Autodesk Fusion 360 part; units mm, degrees
(part 3 of 3)
extrude "Extruir16" cut sketch "Boceto24" against normal blind 2 contours L4 L5 L6 L7 L8 L9 L10 L11 L12 L13 L14 L15 L16 L17 L18 L19 L20 L21 L22 L23 L24 L25 L26 L27 L28 L29 L30 L31 L32 L33 L34 L35 L36 L37 L38 L39 L40 L41 L42 L43 L44 L45 L46 L47 L48 L49 L50 L51 L52 L53 L54 L55 L56 L57 L58 L59 L60 L61 L62 L63 L64 L65 L66 L67 L68 L69 L70 L71 L72 L73 L74 L75 L76 L77 L78 L79 L80 L81 L82 L83 L84 L85 L86 L87 L88 L89 L90 L91 L92 L93 L94 L95 L96 L97 L98 L99 L100 L101 L102 L103 L104 L105 L106 L107 L108 L109 L110 L111 L112 L113 L114 L115 L116 L117 L118 L119 L120 L121 L122 L123 L124 L125 L126 L127 L128 L129 L130 L131 L132 L133 L134 L135 L136 L137 L138 L139 L140 L141 L142 L143 L144 L145 L146 L147 L148 L149 L150 L151 L152 L153 L154 L155 L156 L157 L158 L159 L160 L161 L162 L163 L164 L165 L166 L167 L168 L169 L170 L171 L172 L173 L174 L175 L176 L177 L178 L179 L180 L181 L182 L183 L184 L185 L186 L187 L188 L189 L190 L191 L192 L193 L194 L195 L196 L197 L198 L199 L200 L201 L202 L203 L204 L205 L206 L207 L208 L209 L210 L211 L212 L213 L214 L215 L216 L217 L218 L219 L220 L221 L222 L223 L224 L225 L226 L227 L228 L229 L230 L231 L232 L233 L234 L235 L236 L237 L238 L239 L240 L241 L242 L243 L244 L245 L246 L247 L248 L249 L250 L251 L252 L253 L254 L255 L256 L257 L258 L259 L260 L261 L262 L263 L264 L265 L266 L267 L268 L269 L270 L271 L272 L273 L274 L275 L276 L277 L278 L279 L280 L281 L282 L283 L284 L285 L286 L287 | L288 L289 L290 L291 L292 L293 L294 L295 L296 L297 L298 L299 L300 L301 L302 L303 L304 L305 L306 L307 L308 L309 L310 L311 L312 L313 L314 L315 L316 L317 L318 L319 L320 L321 L322 L323 L324 L325 L326 L327 L328 L329 L330 L331 L332 L333 L334 L335 L336 L337 L338 L339 L340 L341 L342 L343 L344 | L345 L346 L347 L348 L349 L350 L351 L352 L353 L354 L355 L356 L357 L358 L359 L360 L361 L362 L363 L364 L365 L366 L367 L368 L369 L370 L371 L372 L373 L374 L375 L376 L377 L378 L379 L380 L381 L382 L383 L384 L385 L386 L387 L388 L389 L390 L391 L392 L393 L394 L395 L396 L397 L398 L399 L400 L401 L402 L403 L404 L405 L406 L407 L408 L409 L410 L411 L412 L413 L414 L415 L416 L417 L418 L419 L420 L421 L422 L423 L424 L425 L426 L427 L428 L429 L430 L431 L432 L433 L434 L435 L436 L437 L438 L439 L440 L441 L442 L443 L444 L445 L446 L447 | L448 L449 L450 L451 L452 L453 L454 L455 L456 L457 L458 L459 L460 L461 L462 L463 L464 L465 L466 L467 L468 L469 L470 L471 L472 L473 L474 L475 L476 L477 L478 L479 L480 L481 L482 L483 L484 L485 L486 L487 L488 L489 L490 L491 L492 L493 L494 L495 L496 L497 L498 L499 L500 L501 L502 L503 L504 L505 L506 L507 L508 L509 L510 L511 L512 L513 L514 L515 L516 L517 L518 L519 L520 L521 L522 L523 L524 L525 L526 L527 L528 L529 L530 L531 L532 L533 L534 L535 L536 L537 L538 L539 L540 L541 L542 L543 L544 L545 L546 L547 L548 L549 L550 | L551 L552 L553 L554 L555 L556 L557 L558 L560 L561 L562 L563 L564 L565 L566 L567 L569 L570 L571 L572 L573 L575 L576 L577 L579 L580 L581 L583 L584 L585 L586 L587 L588 L589 L590 L591 L592 L593 L594 L595 L596 L597 L598 L599 L600 L601 L602 L603 L604 L605 L606 L607 L608 L609 L610 L611 L612 L613 L614 L616 L617 L618 L619 L620 L621 L622 L623 L625 L626 L627 L628 L629 L630 L631 L632 L634 L635 L636 L637 L638 L639 L640 L641 L642 L643 L688 L690 L691 L692 L696 L697 L698 L699 L700 L701 L702 L703 L704 L705 L707 L708 L709 L710 L711 L712 L714 L715 L716 L717 L718 L719 L720 L721 L722 L723 L725 L726 L727 L728 L729 L730 L731 L732 L733 L734 L735 L738 L739 L740 L741 L742 L743 L744 L745 L746 L747 L748 L749 L750 L751 L752 L753 L754 L755 L756 L757 L758 L759 L760 L761 L762 L763 L765 L766 L767 L769 L770 L771 L773 L774 L775 L776 L777 L778 L779 L781 L783 | L784 L785 L786 L787 L788 L789 L790 L791 L792 L793 L794 L795 L796 L797 L798 L799 L800 L801 L802 L803 L804 L805 L806 L807 L808 L809 L810 L811 L812 L813 L814 L815 L816 L817 L818 L819 L820 L821 L822 L823 L824 L825 L826 L827 L828 L829 L830 L831 L832 L833 L834 L835 L836 L837 L838 L839 bodies 3
ref_plane "PlanoDeObra7" through (97, 32.5, 92.5) normal (1, 0, 0) x (0, 1, 0)
sketch "Boceto29" plane through (0, -6, 0) normal (0, -1, 0) x (1, 0, 0)
  line L0 (25, 74.5) -> (90, 74.5)
  line L1 (90, 74.5) -> (90, 110.5)
  line L2 (90, 110.5) -> (25, 110.5)
  line L3 (25, 110.5) -> (25, 74.5)
  line L4 (32, 82.5) -> (62, 82.5)
  line L5 (62, 82.5) -> (62, 78.5)
  line L6 (62, 78.5) -> (32, 78.5)
  line L7 (32, 78.5) -> (32, 82.5)
  line L8 (19, 74.5) -> (19, 110.5)
  line L9 (74.5, 90.5) -> (84.5, 90.5)
  line L10 (84.5, 90.5) -> (84.5, 84.5)
  line L11 (84.5, 84.5) -> (74.5, 84.5)
  line L12 (74.5, 84.5) -> (74.5, 90.5)
  line L13 (96, 74.5) -> (96, 110.5)
  line L14 (81, 82.5) -> (88, 82.5)
  line L15 (88, 82.5) -> (88, 75.5)
  line L16 (88, 75.5) -> (81, 75.5)
  line L17 (81, 75.5) -> (81, 82.5)
  dimension "d144" = 13
  dimension "d145" = 30
  dimension "d146" = 4
  dimension "d147" = 4
  dimension "d148" = 10
  dimension "d149" = 6
  dimension "d150" = 20
  dimension "d151" = 11.5
  dimension "d152" = 7
  dimension "d153" = 7
  dimension "d154" = 28
  dimension "d155" = 8
  constraint horizontal L4
  constraint vertical L5
  constraint horizontal L6
  constraint vertical L7
  constraint horizontal L9
  constraint vertical L10
  constraint horizontal L11
  constraint vertical L12
  constraint horizontal L14
  constraint vertical L15
  constraint horizontal L16
  constraint vertical L17
  measures "d144" distance of L7 L8
  measures "d145" distance of L4.start L4.end
  measures "d146" distance of L0 L6
  measures "d147" distance of L4.end L5.end
  measures "d148" distance of L9.start L9.end
  measures "d149" distance of L9.start L11.end
  measures "d150" distance of L2 L9
  measures "d151" distance of L10 L13
  measures "d152" distance of L14.start L14.end
  measures "d153" distance of L14.start L16.end
  measures "d154" distance of L2 L14
  measures "d155" distance of L13 L15
extrude "Extruir21" cut sketch "Boceto29" against normal blind 4 contours L4 L5 L6 L7 | L9 L10 L11 L12 | L14 L15 L16 L17 bodies 3
sketch "Boceto30" plane through (0, 71, 0) normal (0, 1, 0) x (-1, 0, 0)
  line L0 (-90, 74.5) -> (-25, 74.5)
  line L1 (-25, 74.5) -> (-25, 110.5)
  line L2 (-25, 110.5) -> (-90, 110.5)
  line L3 (-90, 110.5) -> (-90, 74.5)
  line L4 (-77, 87.5) -> (-27, 87.5)
  line L5 (-27, 87.5) -> (-27, 71.5)
  line L6 (-27, 71.5) -> (-77, 71.5)
  line L7 (-77, 71.5) -> (-77, 87.5)
  line L8 (-19, 110.5) -> (-19, 74.5)
  dimension "d158" = 8
  dimension "d160" = 50
  dimension "d161" = 16
  dimension "d198" = 23
  constraint horizontal L4
  constraint vertical L5
  constraint horizontal L6
  constraint vertical L7
  measures "d158" distance of L5 L8
  measures "d160" distance of L4.start L4.end
  measures "d161" distance of L4.start L6.end
  measures "d198" distance of L2 L4
sketch "Boceto39" plane through (0, 0, 74.5) normal (0, 0, -1) x (1, 0, 0)
  arc A0 (90, -69) -> (94, -65) centre (90, -65) ccw
  line L0 (90, -69) -> (25, -69)
  arc A1 (21, -65) -> (25, -69) centre (25, -65) ccw
  line L1 (21, -65) -> (21, 0)
  arc A2 (25, 4) -> (21, 0) centre (25, 0) ccw
  line L2 (25, 4) -> (90, 4)
  arc A3 (94, 0) -> (90, 4) centre (90, 0) ccw
  line L3 (94, 0) -> (94, -65)
  arc A4 (90, -71) -> (96, -65) centre (90, -65) ccw
  line L4 (96, -65) -> (96, 0)
  arc A5 (96, 0) -> (90, 6) centre (90, 0) ccw
  line L5 (90, 6) -> (25, 6)
  arc A6 (25, 6) -> (19, 0) centre (25, 0) ccw
  line L6 (19, 0) -> (19, -65)
  arc A7 (19, -65) -> (25, -71) centre (25, -65) ccw
  line L7 (25, -71) -> (90, -71)
extrude "Extruir32" cut sketch "Boceto39" along normal blind 4 bodies 2
extrude "Extruir33" add 1 faces at (46.6667, -4.6667, 74.5) along direction (0, 0, -1) blind 4 on bodies 3 bodies 2 3
ref_plane "PlanoDeObra8" through (97, 32.5, 90.5) normal (1, 0, 0) x (0, 1, 0)
sketch "Boceto40" plane through (97, 0, 0) normal (1, 0, 0) x (0, 1, 0)
  line L0 (17, 94.5) -> (52, 94.5)
  line L1 (52, 94.5) -> (52, 76.5)
  line L2 (47, 71.5) -> (22, 71.5)
  line L3 (17, 76.5) -> (17, 94.5)
  line L4 (0, 110.5) -> (65, 110.5)
  line L5 (-6, 74.5) -> (-6, 110.5)
  line L6 (17, 80.5) -> (22, 80.5)
  line L7 (22, 80.5) -> (22, 71.5)
  line L8 (17, 76.5) -> (17, 80.5)
  line L9 (47, 80.5) -> (52, 80.5)
  line L10 (52, 80.5) -> (52, 76.5)
  line L11 (47, 71.5) -> (47, 80.5)
  arc A0 (17, 76.5) -> (22, 71.5) centre (22, 76.5) ccw
  arc A1 (47, 71.5) -> (52, 76.5) centre (47, 76.5) ccw
  circle A2 centre (19.5, 77) radius 1.5
  circle A3 centre (49.5, 77) radius 1.5
  arc A4 (47, 71.5) -> (52, 76.5) centre (47, 76.5) ccw
  arc A5 (47, 70.5) -> (53, 76.5) centre (47, 76.5) ccw
  line L12 (53, 95.5) -> (53, 76.5)
  line L13 (16, 95.5) -> (53, 95.5)
  line L14 (16, 76.5) -> (16, 95.5)
  arc A6 (16, 76.5) -> (22, 70.5) centre (22, 76.5) ccw
  line L15 (47, 70.5) -> (22, 70.5)
  arc A7 (17, 76.5) -> (22, 71.5) centre (22, 76.5) ccw
  point P0 (17, 71.5)
  dimension "d204" = 35
  dimension "d205" = 23
  dimension "d206" = 16
  dimension "d207" = 23
  dimension "d209" = 5
  dimension "d210" = 5
  dimension "d211" = 30
  dimension "d212" = 30
  dimension "d213" = 5
  dimension "d214" = 5
  dimension "d215" = 3
  dimension "d216" = 3.5
  dimension "d217" = 2.5
  dimension "d218" = 3
  dimension "d219" = 3.5
  dimension "d220" = 2.5
  dimension "d221" = 5
  dimension "d222" = -1
  dimension "d223" = 5
  constraint horizontal L0
  constraint vertical L1
  constraint horizontal L2
  constraint vertical L3
  constraint horizontal L6
  constraint vertical L7
  constraint vertical L8
  constraint coincident L2 L7.end
  constraint coincident L3 L6.start
  constraint horizontal L9
  constraint vertical L10
  constraint vertical L11
  constraint coincident P0 L2
  constraint coincident P0 L3
  constraint tangent L2 A0
  constraint tangent L3 A0
  constraint tangent L10 A1
  constraint coincident L2.start L11.start
  constraint tangent L1 A4
  constraint tangent L2 A4
  constraint tangent L8 A7
  constraint coincident L2.end L7.end
  measures "d204" distance of L0.start L0.end
  measures "d205" distance of L0.start P0
  measures "d206" distance of L0 L4
  measures "d207" distance of L3 L5
  measures "d209" distance of L6.start L6.end
  measures "d210" distance of L9.start L9.end
  measures "d211" distance of L4 L6
  measures "d212" distance of L4 L9
  measures "d213" radius of A0
  measures "d214" radius of A1
  measures "d215" diameter of A2
  measures "d216" distance of L6 A2.centre
  measures "d217" distance of L8 A2.centre
  measures "d218" diameter of A3
  measures "d219" distance of L9 A3.centre
  measures "d220" distance of L1 A3.centre
  measures "d221" radius of A4
  measures "d223" radius of A7
extrude "Extruir34" add sketch "Boceto40" along normal blind 2.2 separate body contours L3 L6 L7 L8 A0 A7 | L1 L9 L10 L11 A1 A4 | A5 L12 L13 L14 A6 L15 makes body 5
sketch "Boceto41" plane through (99.2, 0, 0) normal (1, 0, 0) x (0, 1, 0)
  circle A0 centre (49.5, 77) radius 1.5
  circle A1 centre (19.5, 77) radius 1.5
  line L0 (22, 80.5) -> (17, 80.5)
  line L1 (17, 80.5) -> (17, 94.5)
  line L2 (17, 94.5) -> (52, 94.5)
  line L3 (52, 94.5) -> (52, 80.5)
  line L4 (52, 80.5) -> (47, 80.5)
  line L5 (47, 80.5) -> (47, 71.5)
  line L6 (47, 71.5) -> (22, 71.5)
  line L7 (22, 71.5) -> (22, 80.5)
  arc A2 (16, 76.5) -> (22, 70.5) centre (22, 76.5) ccw
  line L8 (22, 70.5) -> (47, 70.5)
  arc A3 (47, 70.5) -> (53, 76.5) centre (47, 76.5) ccw
  line L9 (53, 76.5) -> (53, 95.5)
  line L10 (53, 95.5) -> (16, 95.5)
  line L11 (16, 95.5) -> (16, 76.5)
  line L12 (16, 95.5) -> (53, 95.5)
  line L13 (53, 95.5) -> (53, 76.5)
  line L14 (47, 70.5) -> (22, 70.5)
  line L15 (16, 76.5) -> (16, 95.5)
  arc A4 (16, 76.5) -> (22, 70.5) centre (22, 76.5) ccw
  arc A5 (47, 70.5) -> (53, 76.5) centre (47, 76.5) ccw
  line L16 (52, 94.5) -> (52, 76.5)
  arc A6 (47, 71.5) -> (52, 76.5) centre (47, 76.5) ccw
  line L17 (47, 71.5) -> (22, 71.5)
  arc A7 (17, 76.5) -> (22, 71.5) centre (22, 76.5) ccw
  line L18 (17, 76.5) -> (17, 94.5)
  line L19 (17, 94.5) -> (52, 94.5)
  dimension "d226" = 6
  dimension "d227" = 6
  dimension "d228" = 1
  constraint horizontal L12
  constraint vertical L13
  constraint horizontal L14
  constraint vertical L15
  constraint coincident L10.end L11.start
  constraint tangent L14 A4
  constraint tangent L15 A4
  constraint tangent L13 A5
  constraint tangent L14 A5
  measures "d226" radius of A4
  measures "d227" radius of A5
extrude "Extruir35" add sketch "Boceto41" along normal blind 47.2 contours A2 L8 A3 L9 L10 L11 L12 L13 L14 L15 A4 A5 bodies 5
sketch "Boceto42" plane through (146.4, 0, 0) normal (1, 0, 0) x (0, 1, 0)
  arc A0 (17, 76.5) -> (22, 71.5) centre (22, 76.5) ccw
  line L0 (17, 76.5) -> (17, 94.5)
  line L1 (17, 94.5) -> (52, 94.5)
  line L2 (52, 94.5) -> (52, 76.5)
  arc A1 (47, 71.5) -> (52, 76.5) centre (47, 76.5) ccw
  line L3 (47, 71.5) -> (22, 71.5)
  arc A2 (16, 76.5) -> (22, 70.5) centre (22, 76.5) ccw
  line L4 (22, 70.5) -> (47, 70.5)
  arc A3 (47, 70.5) -> (53, 76.5) centre (47, 76.5) ccw
  line L5 (53, 76.5) -> (53, 95.5)
  line L6 (53, 95.5) -> (16, 95.5)
  line L7 (16, 95.5) -> (16, 76.5)
  line L8 (16, 95.5) -> (53, 95.5)
  line L9 (53, 95.5) -> (53, 76.5)
  line L10 (47, 70.5) -> (22, 70.5)
  line L11 (16, 76.5) -> (16, 95.5)
  arc A4 (16, 76.5) -> (22, 70.5) centre (22, 76.5) ccw
  arc A5 (47, 70.5) -> (53, 76.5) centre (47, 76.5) ccw
  dimension "d231" = 6
  dimension "d232" = 6
  constraint horizontal L8
  constraint vertical L9
  constraint horizontal L10
  constraint vertical L11
  constraint coincident L6.end L7.start
  constraint tangent L10 A4
  constraint tangent L11 A4
  constraint tangent L9 A5
  constraint tangent L10 A5
  measures "d231" radius of A4
  measures "d232" radius of A5
extrude "Extruir36" add sketch "Boceto42" along normal blind 1 contours A0 L0 L1 L2 A1 L3 | A2 L4 A3 L5 L6 L7 L8 L9 L10 L11 A4 A5 bodies 5
extrude "Extruir15" cut sketch "Boceto22" against normal blind 5 contours L4 L5 L6 L7 A5 A6 A7 A8 | A4 bodies 4
extrude "Extruir37" add 4 faces at (91.1802, 66.1672, 72.5) (24.2816, 64.7922, 72.5) (91.6771, -1.4276, 72.5) (24.2881, -3.0007, 72.5) along direction (0, 0, 1) blind 1 on bodies 2 bodies 2
sketch "Boceto44" plane through (0, 0, 73.5) normal (0, 0, 1) x (-1, 0, 0)
  line L0 (-21, -65) -> (-21, 0)
  arc A0 (-21, 0) -> (-25, 4) centre (-25, 0) ccw
  line L1 (-25, 4) -> (-90, 4)
  arc A1 (-90, 4) -> (-94, 0) centre (-90, 0) ccw
  line L2 (-94, 0) -> (-94, -65)
  arc A2 (-94, -65) -> (-90, -69) centre (-90, -65) ccw
  line L3 (-90, -69) -> (-25, -69)
  arc A3 (-25, -69) -> (-21, -65) centre (-25, -65) ccw
  line L4 (-29.1428, -48.4634) -> (-65.8572, -48.4634)
  line L5 (-65.8572, -48.4634) -> (-65.8572, -16.5366)
  line L6 (-65.8572, -16.5366) -> (-29.1428, -16.5366)
  line L7 (-29.1428, -16.5366) -> (-29.1428, -48.4634)
  line L8 (-94, -2) -> (-88, -2)
  line L9 (-88, -2) -> (-88, 4)
  line L10 (-88, 4) -> (-90, 4)
  line L11 (-94, 0) -> (-94, -2)
  arc A4 (-90, 4) -> (-94, 0) centre (-90, 0) ccw
  circle A5 centre (-90.6, 0.6) radius 1.5
  line L12 (-21, -2) -> (-27, -2)
  line L13 (-27, -2) -> (-27, 4)
  line L14 (-27, 4) -> (-25, 4)
  line L15 (-21, 0) -> (-21, -2)
  arc A6 (-21, 0) -> (-25, 4) centre (-25, 0) ccw
  circle A7 centre (-24.4, 0.6) radius 1.5
  line L16 (-21, -63) -> (-27, -63)
  line L17 (-27, -63) -> (-27, -69)
  line L18 (-27, -69) -> (-25, -69)
  line L19 (-21, -65) -> (-21, -63)
  arc A8 (-25, -69) -> (-21, -65) centre (-25, -65) ccw
  circle A9 centre (-24.4, -65.6) radius 1.5
  line L20 (-94, -63) -> (-88, -63)
  line L21 (-88, -63) -> (-88, -69)
  line L22 (-88, -69) -> (-90, -69)
  line L23 (-94, -65) -> (-94, -63)
  arc A10 (-94, -65) -> (-90, -69) centre (-90, -65) ccw
  circle A11 centre (-90.6, -65.6) radius 1.5
  dimension "d238" = 6
  dimension "d239" = 6
  dimension "d240" = 4
  dimension "d241" = 3
  dimension "d242" = 2.6
  dimension "d243" = 2.6
  dimension "d244" = 6
  dimension "d245" = 6
  dimension "d246" = 4
  dimension "d247" = 3
  dimension "d248" = 2.6
  dimension "d249" = 2.6
  dimension "d250" = 6
  dimension "d251" = 6
  dimension "d252" = 4
  dimension "d253" = 3
  dimension "d254" = 2.6
  dimension "d255" = 2.6
  dimension "d256" = 6
  dimension "d257" = 6
  dimension "d258" = 4
  dimension "d259" = 3
  dimension "d260" = 2.6
  dimension "d261" = 2.6
  constraint horizontal L8
  constraint vertical L9
  constraint horizontal L10
  constraint vertical L11
  constraint coincident L1 L9.end
  constraint coincident L2 L8.start
  constraint tangent L10 A4
  constraint tangent L11 A4
  constraint horizontal L12
  constraint vertical L13
  constraint horizontal L14
  constraint vertical L15
  constraint coincident L1 L13.end
  constraint coincident L0 L12.start
  constraint tangent L14 A6
  constraint tangent L15 A6
  constraint horizontal L16
  constraint vertical L17
  constraint horizontal L18
  constraint vertical L19
  constraint coincident L3 L17.end
  constraint coincident L0 L16.start
  constraint tangent L18 A8
  constraint tangent L19 A8
  constraint horizontal L20
  constraint vertical L21
  constraint horizontal L22
  constraint vertical L23
  constraint coincident L3 L21.end
  constraint coincident L2 L20.start
  constraint tangent L22 A10
  constraint tangent L23 A10
  measures "d238" distance of L8.start L8.end
  measures "d239" distance of L8.end L9.end
  measures "d240" radius of A4
  measures "d241" diameter of A5
  measures "d242" distance of L9 A5.centre
  measures "d243" distance of L8 A5.centre
  measures "d244" distance of L12.start L12.end
  measures "d245" distance of L12.end L13.end
  measures "d246" radius of A6
  measures "d247" diameter of A7
  measures "d248" distance of L13 A7.centre
  measures "d249" distance of L12 A7.centre
  measures "d250" distance of L16.start L16.end
  measures "d251" distance of L16.end L17.end
  measures "d252" radius of A8
  measures "d253" diameter of A9
  measures "d254" distance of L17 A9.centre
  measures "d255" distance of L16 A9.centre
  measures "d256" distance of L20.start L20.end
  measures "d257" distance of L20.end L21.end
  measures "d258" radius of A10
  measures "d259" diameter of A11
  measures "d260" distance of L20 A11.centre
  measures "d261" distance of L21 A11.centre
extrude "Extruir38" add sketch "Boceto44" along normal blind 2 contours L0 L3 A3 L16 L17 L18 L19 A8 | L0 A0 L1 L12 L13 L14 L15 A6 | L2 A2 L3 L20 L21 L22 L23 A10 | L1 A1 L2 L8 L9 L10 L11 A4 bodies 2
ref_plane "PlanoDeObra9" through (24, -1, 76.5) normal (0, 0, 1) x (-1, 0, 0)
sketch "Boceto45" plane through (0, 0, 76.5) normal (0, 0, 1) x (1, 0, 0)
  line L0 (27, -4) -> (25, -4)
  line L1 (21, 0) -> (21, 2)
  line L2 (21, 2) -> (27, 2)
  line L3 (27, 2) -> (27, -4)
  arc A0 (21, 0) -> (25, -4) centre (25, 0) ccw
  circle A1 centre (24.4, -0.6) radius 1.5
  line L4 (27, 63) -> (21, 63)
  line L5 (21, 63) -> (21, 65)
  line L6 (25, 69) -> (27, 69)
  line L7 (27, 69) -> (27, 63)
  arc A2 (25, 69) -> (21, 65) centre (25, 65) ccw
  circle A3 centre (24.4, 65.6) radius 1.4976
  line L8 (94, 63) -> (88, 63)
  line L9 (88, 63) -> (88, 69)
  line L10 (88, 69) -> (90, 69)
  line L11 (94, 65) -> (94, 63)
  arc A4 (94, 65) -> (90, 69) centre (90, 65) ccw
  circle A5 centre (90.6, 65.6) radius 1.5
  line L12 (88, -4) -> (90, -4)
  line L13 (94, 0) -> (94, 2)
  line L14 (94, 2) -> (88, 2)
  line L15 (88, 2) -> (88, -4)
  arc A6 (90, -4) -> (94, 0) centre (90, 0) ccw
  circle A7 centre (90.6, -0.6) radius 1.5
  dimension "d265" = 4
  dimension "d266" = 3
  dimension "d267" = 2.6
  dimension "d268" = 2.6
  dimension "d269" = 4
  dimension "d270" = 2.6
  dimension "d271" = 2.6
  dimension "d272" = 4
  dimension "d273" = 2.6
  dimension "d274" = 2.6
  dimension "d275" = 3
  dimension "d276" = 4
  dimension "d277" = 2.6
  dimension "d278" = 2.6
  dimension "d279" = 3
  constraint horizontal L0
  constraint vertical L1
  constraint horizontal L2
  constraint vertical L3
  constraint tangent L0 A0
  constraint tangent L1 A0
  constraint horizontal L4
  constraint vertical L5
  constraint horizontal L6
  constraint vertical L7
  constraint tangent L5 A2
  constraint tangent L6 A2
  constraint horizontal L8
  constraint vertical L9
  constraint horizontal L10
  constraint vertical L11
  constraint tangent L10 A4
  constraint tangent L11 A4
  constraint horizontal L12
  constraint vertical L13
  constraint horizontal L14
  constraint vertical L15
  constraint tangent L12 A6
  constraint tangent L13 A6
  measures "d265" radius of A0
  measures "d266" diameter of A1
  measures "d267" distance of L3 A1.centre
  measures "d268" distance of L2 A1.centre
  measures "d269" radius of A2
  measures "d270" distance of L4 A3.centre
  measures "d271" distance of L7 A3.centre
  measures "d272" radius of A4
  measures "d273" distance of L8 A5.centre
  measures "d274" distance of L9 A5.centre
  measures "d275" diameter of A5
  measures "d276" radius of A6
  measures "d277" distance of L15 A7.centre
  measures "d278" distance of L14 A7.centre
  measures "d279" diameter of A7
extrude "Extruir39" add sketch "Boceto45" along normal blind 2 bodies 2
